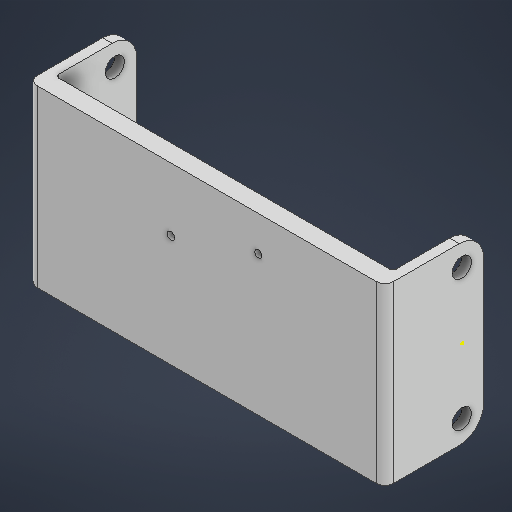
# Autodesk Inventor part: LaserBeslag
Saved by Autodesk Inventor 2026.2 (Build 302298010, 298A)
## iProperties
Created: 2026-04-22
Part Number: LaserBeslag
Material: Generic
Document SubType Name: Modeling
Designer: frede
Density: 1 g/cm^3
Appearance: Default
Author: frede
Autodesk Inventor part; units mm, degrees
ref_plane "YZ Plane" through (0, 0, 0) normal (1, 0, 0) x (0, 1, 0)
ref_plane "XZ Plane" through (0, 0, 0) normal (0, 1, 0) x (-1, 0, 0)
ref_plane "XY Plane" through (0, 0, 0) normal (0, 0, 1) x (1, 0, 0)
sketch "Sketch1" plane through (0, 0, 0) normal (1, 0, 0) x (0, 1, 0)
  circle A0 centre (-37.5, 0) radius 5.5
  circle A1 centre (37.5, 0) radius 5.5
  line L0 (-50, 44) -> (50, 44)
  line L1 (50, 44) -> (50, -12.5)
  line L2 (50, -12.5) -> (-50, -12.5)
  line L3 (-50, -12.5) -> (-50, 44)
  point P0 (0, 0)
  dimension "d0" = 11
  dimension "d1" = 11
  dimension "d2" = 100
  dimension "d3" = 56.5
  constraints: 8 end point, 2 centre point, 2 parallel, 1 horizontal, 1 perpendicular
  measures "d0" diameter of A0
  measures "d1" diameter of A1
  measures "d2" distance of L1.end L2.end
  measures "d3" distance of L0.end L1.end
extrude "Extrusion1" add sketch "Sketch1" along normal blind 204
sketch "Sketch2" plane through (0, -50, -12.5) normal (0, -1, 0) x (1, 0, 0)
  line L0 (204, 0) -> (204, 56.5) projected
  line L1 (0, 0) -> (204, 0)
  line L2 (204, 0) -> (204, 56.5)
  line L3 (204, 56.5) -> (0, 56.5)
  line L4 (0, 56.5) -> (0, 0)
  line L5 (5.5, 0) -> (198.5, 0)
  line L6 (198.5, 0) -> (198.5, 46.5)
  line L7 (198.5, 46.5) -> (5.5, 46.5)
  line L8 (5.5, 46.5) -> (5.5, 0)
  point P0 (0, 12.5)
  point P1 (198.5, 0)
  dimension "d6" = 204
  dimension "d7" = 193
  dimension "d8" = 46.5
  dimension "d9" = 5.5
  constraints: 16 end point, 4 parallel, 2 horizontal, 2 perpendicular, 1 point on line
  measures "d6" distance between parallel lines of L0 L4
  measures "d7" distance of L7.end L6.end
  measures "d8" distance of L6.end L5.end
  measures "d9" distance between parallel lines of L4 L8
extrude "Extrusion2" cut sketch "Sketch2" against normal up to surface (100 mm away) contours L1 L8 L7 L6
sketch "Sketch3" plane through (204, 0, 0) normal (1, 0, 0) x (0, 0, -1)
  point P0 (0, 0)
fillet "Fillet1" radius 14 4 edges at (201.25, 50, -12.5) (201.25, -50, -12.5) (2.75, 50, -12.5) (2.75, -50, -12.5)
fillet "Fillet2" radius 2 2 edges at (198.5, 0, 34) (5.5, 0, 34)
fillet "Fillet3" radius 5 2 edges at (204, 0, 44) (0, 0, 44)
sketch "Sketch4" plane through (196.5, -50, 34) normal (0, 0, -1) x (-1, 0, 0)
  line L0 (0, 100) -> (189, 100) projected
  line L1 (58.5, 100) -> (118.5, 100)
  line L2 (118.5, 100) -> (118.5, 58)
  line L3 (118.5, 58) -> (58.5, 58)
  line L4 (58.5, 58) -> (58.5, 100)
  circle A0 centre (64.9, 80) radius 4
  circle A1 centre (114.9, 64) radius 4
  line L5 (-7.5, 14) -> (-7.5, 86) projected
  line L6 (94.5, 58) -> (94.5, 100)
  line L7 (196.5, 14) -> (196.5, 86) projected
  point P0 (196.5, 50)
  dimension "d15" = 60
  dimension "d16" = 42
  dimension "d17" = 8
  dimension "d19" = 6.4
  dimension "d20" = 8
  dimension "d22" = 6
  dimension "d24" = 36
  dimension "d25" = 102
  dimension "d26" = 204
  dimension "d34" = 16
  dimension "d36" = 50
  constraints: 10 end point, 3 point on line, 2 centre point, 2 parallel, 2 perpendicular, 1 horizontal
  measures "d15" distance of L2.end L3.end
  measures "d16" distance of L1.end L2.end
  measures "d17" diameter of A0
  measures "d19" distance from line of L4 A0.centre
  measures "d20" diameter of A1
  measures "d22" distance from line of L3 A1.centre
  measures "d24" distance between parallel lines of L4 L6
  measures "d25" distance between parallel lines of L6 L5
  measures "d26" distance between parallel lines of L7 L5
  measures "d34" vertical distance of A1.centre A0.centre
  measures "d36" horizontal distance of A1.centre A0.centre
extrude "Extrusion3" cut sketch "Sketch4" against normal blind 4 contours A1 L2 | L2 A1 | A0
sketch "Sketch5" plane through (131.6, 30, 38) normal (0, 0, -1) x (-1, 0, 0)
  circle A0 centre (0, 0) radius 4 projected
  circle A1 centre (50, -16) radius 4 projected
  circle A2 centre (0, 0) radius 2.125
  circle A3 centre (50, -16) radius 2.125
  point P0 (131.6, -30)
  dimension "d29" = 4.25
  dimension "d30" = 4.25
  constraints: 4 coincident, 2 centre point
  measures "d29" diameter of A2
  measures "d30" diameter of A3
extrude "Extrusion4" cut sketch "Sketch5" against normal blind 6 contours A2 | A3
equation "\"d9\" = -0.5 * d7 + 0.5 * d6"
equation "\"d25\" = 0.5 * d26"
body "Solid1"
